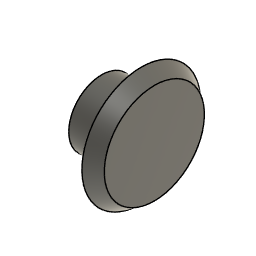
Four-Cylinder Engine_ (Autodesk Fusion 360 archive; units mm, degrees)
design "Rivet"
Autodesk Fusion 360 part; units mm, degrees
sketch "Sketch1" plane through (0, 0, 0) normal (0, 1, 0) x (1, 0, 0)
  line L0 (0, 0) -> (101.6, 0)
  line L1 (101.6, 0) -> (101.6, -96.5147)
  line L2 (101.6, -96.5147) -> (76.2, -114.3)
  line L3 (76.2, -114.3) -> (76.2, -63.5)
  line L4 (76.2, -63.5) -> (0, -63.5)
  line L5 (0, -63.5) -> (0, 0)
  dimension "d1" = 101.6
  dimension "d2" = 76.2
  dimension "d3" = 55
  dimension "d4" = 127
  dimension "d5" = 228.6
  constraint coincident L0.start L5.end
  constraint horizontal L0
  constraint perpendicular L0 L3
  constraint perpendicular L3 L4
  constraint vertical L1
  constraint vertical L5
  measures "d1" distance of L0.start L0.end
  measures "d2" distance of L3.end L4.end
  measures "d3" angle of L2 L3
revolve "Revolve1" add sketch "Sketch1" angle 360 about axis through (0, 0, 0) along (1, 0, 0)

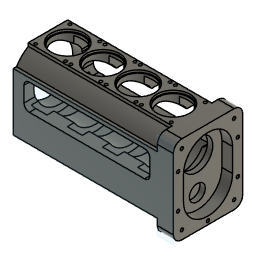
design "Engine Block"
Autodesk Fusion 360 part; units mm, degrees
sketch "Sketch1" plane through (0, 0, 0) normal (1, 0, 0) x (0, 1, 0)
  line L0 (-825.5, 1041.4) -> (825.5, 1041.4)
  line L1 (825.5, 1041.4) -> (825.5, -1041.4)
  line L2 (825.5, -1041.4) -> (-825.5, -1041.4)
  line L3 (-825.5, -1041.4) -> (-825.5, 1041.4)
  line L4 (-825.5, 1041.4) -> (825.5, -1041.4) construction
  line L5 (825.5, 1041.4) -> (-825.5, -1041.4) construction
  dimension "d1" = 1651
  dimension "d2" = 2082.8
  constraint horizontal L0
  constraint perpendicular L0 L1
  constraint parallel L0 L2
  constraint parallel L1 L3
  constraint coincident L4 origin
  constraint coincident L5 origin
  measures "d1" distance of L0.start L0.end
  measures "d2" distance of L0.end L1.end
extrude "Extrude1" add sketch "Sketch1" along normal mid plane 3810
sketch "Sketch2" plane through (1905, 0, 0) normal (1, 0, 0) x (0, 1, 0)
  line L0 (-825.5, -1041.4) -> (825.5, -1041.4)
  line L1 (825.5, -1041.4) -> (825.5, 1041.4)
  line L2 (825.5, 1041.4) -> (-825.5, 1041.4)
  line L3 (-825.5, 1041.4) -> (-825.5, -1041.4)
  circle A0 centre (0, 279.4) radius 368.3
  dimension "d5" = 736.6
  dimension "d6" = 279.4
  constraint vertical origin A0.centre
  measures "d5" diameter of A0
  measures "d6" distance of origin A0.centre
extrude "Extrude2" cut sketch "Sketch2" against normal through all contours A0
sketch "Sketch3" plane through (1905, 0, 0) normal (1, 0, 0) x (0, 1, 0)
  circle A0 centre (0, 279.4) radius 368.3
  line L0 (-825.5, -1041.4) -> (825.5, -1041.4)
  line L1 (825.5, -1041.4) -> (825.5, 1041.4)
  line L2 (825.5, 1041.4) -> (-825.5, 1041.4)
  line L3 (-825.5, 1041.4) -> (-825.5, -1041.4)
  line L4 (-584.2, 279.4) -> (-584.2, -279.4)
  arc A1 (-584.2, -279.4) -> (584.2, -279.4) centre (0, -279.4) ccw
  line L5 (584.2, -279.4) -> (584.2, 279.4)
  arc A2 (584.2, 279.4) -> (-584.2, 279.4) centre (0, 279.4) ccw
  line L6 (0, 279.4) -> (0, -279.4) construction
  dimension "d8" = 584.2
  dimension "d9" = 558.8
  constraint tangent L4 A1
  constraint tangent A1 L5
  constraint parallel L4 L5
  constraint tangent L5 A2
  constraint tangent L4 A2
  constraint vertical L6
  constraint coincident A0.centre A2.centre
  measures "d8" radius of A2
  measures "d9" distance of A0.centre A1.centre
extrude "Extrude3" cut sketch "Sketch3" against normal blind 254 contours L4 A1 L5 A2
sketch "Sketch4" plane through (-1905, 0, 0) normal (-1, 0, 0) x (0, -1, 0)
  circle A0 centre (0, 279.4) radius 368.3
  line L0 (-825.5, -1041.4) -> (825.5, -1041.4)
  line L1 (825.5, -1041.4) -> (825.5, 1041.4)
  line L2 (825.5, 1041.4) -> (-825.5, 1041.4)
  line L3 (-825.5, 1041.4) -> (-825.5, -1041.4)
  circle A1 centre (0, 279.4) radius 590.55
  dimension "d12" = 1181.1
  constraint concentric A0 A1
  measures "d12" diameter of A1
extrude "Extrude4" cut sketch "Sketch4" against normal blind 3429 contours A1
sketch "Sketch5" plane through (-1905, 0, 0) normal (-1, 0, 0) x (0, -1, 0)
  circle A0 centre (0, 279.4) radius 590.55
  line L0 (-825.5, -1041.4) -> (825.5, -1041.4)
  line L1 (825.5, -1041.4) -> (825.5, 1041.4)
  line L2 (825.5, 1041.4) -> (-825.5, 1041.4)
  line L3 (-825.5, 1041.4) -> (-825.5, -1041.4)
  line L4 (-419.1, -1041.4) -> (-749.3, -685.8)
  line L5 (-749.3, -685.8) -> (-825.5, -685.8)
  line L6 (-825.5, 685.8) -> (-749.3, 685.8)
  line L7 (-469.9, 965.2) -> (-469.9, 1041.4)
  line L8 (0, 0) -> (0, 1263.6507) construction
  arc A1 (-469.9, 965.2) -> (-749.3, 685.8) centre (-15.1369, 231.0369) ccw
  line L9 (825.5, 685.8) -> (749.3, 685.8)
  arc A2 (749.3, 685.8) -> (469.9, 965.2) centre (15.1369, 231.0369) ccw
  line L10 (469.9, 965.2) -> (469.9, 1041.4)
  line L11 (749.3, -685.8) -> (825.5, -685.8)
  line L12 (419.1, -1041.4) -> (749.3, -685.8)
  dimension "d15" = 76.2
  dimension "d16" = 76.2
  dimension "d17" = 355.6
  dimension "d18" = 355.6
  dimension "d20" = 863.6
  dimension "d21" = 76.2
  dimension "d22" = 355.6
  dimension "d23" = 406.4
  constraint coincident L0 L4.start
  constraint coincident L3 L5.end
  constraint perpendicular L3 L5
  constraint coincident L3 L6.start
  constraint perpendicular L3 L6
  constraint coincident L2 L7.end
  constraint perpendicular L2 L7
  constraint coincident L8.start origin
  constraint perpendicular L2 L8
  constraint symmetric L4.start L8 L12.start
  constraint symmetric L4.end L8 L11.start
  constraint symmetric L5.end L8 L11.end
  constraint symmetric L6.start L8 L9.start
  constraint symmetric L6.end L8 L9.end
  constraint symmetric L7.start L8 A2.end
  constraint symmetric L7.end L8 L10.end
  constraint symmetric L8 A1 A2
  measures "d15" distance of L7.start L7.end
  measures "d16" distance of L6.start L6.end
  measures "d17" distance of L2.end L7.end
  measures "d18" distance of L2.end L6.start
  measures "d20" radius of A1
  measures "d21" distance of L4.end L5.end
  measures "d22" distance of L0.start L5.end
  measures "d23" distance of L0.start L4.start
extrude "Extrude5" cut sketch "Sketch5" against normal blind 3429 contours L0 L3 L4 L5 | L0 L1 L11 L12 | L2 L3 L6 L7 A1 | L1 L2 L9 A2 L10
sketch "Sketch6" plane through (0, 0, 1041.4) normal (0, 0, 1) x (-1, 0, 0)
  line L0 (-1524, 469.9) -> (-1524, 825.5)
  line L1 (-1524, 825.5) -> (-1905, 825.5)
  line L2 (-1905, 825.5) -> (-1905, -825.5)
  line L3 (-1905, -825.5) -> (-1524, -825.5)
  line L4 (-1524, -825.5) -> (-1524, -469.9)
  line L5 (-1524, -469.9) -> (1905, -469.9)
  line L6 (1905, -469.9) -> (1905, 469.9)
  line L7 (1905, 469.9) -> (-1524, 469.9)
  circle A0 centre (-1079.5, 0) radius 368.3
  circle A1 centre (-241.3, 0) radius 368.3
  circle A2 centre (596.9, 0) radius 368.3
  circle A3 centre (1435.1, 0) radius 368.3
  dimension "d26" = 736.6
  dimension "d27" = 825.5
  dimension "d30" = 2514.6
  dimension "d31" = 0
  constraint horizontal origin A0.centre
  measures "d26" diameter of A0
  measures "d27" distance of L2 A0.centre
extrude "Extrude6" cut sketch "Sketch6" against normal blind 762 contours A0 | A1 | A2 | A3
sketch "Sketch7" plane through (0, 0, 1041.4) normal (0, 0, 1) x (-1, 0, 0)
  circle A0 centre (596.9, 0) radius 368.3
  circle A1 centre (-241.3, 0) radius 368.3
  circle A2 centre (1435.1, 0) radius 368.3
  circle A3 centre (-1079.5, 0) radius 368.3
  line L0 (-1524, 469.9) -> (-1524, 825.5)
  line L1 (-1524, 825.5) -> (-1905, 825.5)
  line L2 (-1905, 825.5) -> (-1905, -825.5)
  line L3 (-1905, -825.5) -> (-1524, -825.5)
  line L4 (-1524, -825.5) -> (-1524, -469.9)
  line L5 (-1524, -469.9) -> (1905, -469.9)
  line L6 (1905, -469.9) -> (1905, 469.9)
  line L7 (1905, 469.9) -> (-1524, 469.9)
  circle A4 centre (-1079.5, 0) radius 393.7
  circle A5 centre (-241.3, 0) radius 393.7
  circle A6 centre (596.9, 0) radius 393.7
  circle A7 centre (1435.1, 0) radius 393.7
  dimension "d34" = 787.4
  dimension "d37" = 2514.6
  dimension "d38" = 0
  constraint concentric A3 A4
  measures "d34" diameter of A4
extrude "Extrude7" cut sketch "Sketch7" against normal blind 50.8 contours A4 | A5 | A6 | A7
sketch "Sketch8" plane through (0, -825.5, 0) normal (0, -1, 0) x (1, 0, 0)
  line L0 (1524, 1041.4) -> (1524, 685.8)
  line L1 (1524, 685.8) -> (-1905, 685.8)
  line L2 (-1905, 685.8) -> (-1905, -685.8)
  line L3 (-1905, -685.8) -> (1524, -685.8)
  line L4 (1524, -685.8) -> (1524, -1041.4)
  line L5 (1524, -1041.4) -> (1905, -1041.4)
  line L6 (1905, -1041.4) -> (1905, 1041.4)
  line L7 (1905, 1041.4) -> (1524, 1041.4)
sketch "Sketch9" plane through (0, 0, 0) normal (0, 1, 0) x (1, 0, 0)
  line L0 (-2322.3907, -279.4) -> (2570.9498, -279.4) construction
  line L1 (901.7, -1016) -> (1257.3, -1016)
  line L2 (1257.3, -1016) -> (1257.3, -279.4)
  line L3 (1257.3, -279.4) -> (901.7, -279.4)
  line L4 (901.7, -279.4) -> (901.7, -1016)
  point P0 (1905, -1041.4)
  dimension "d41" = 355.6
  dimension "d42" = 647.7
  dimension "d43" = 1473.2
  dimension "d44" = 279.4
  constraint horizontal L0
  constraint horizontal L1
  constraint vertical L2
  constraint horizontal L3
  constraint vertical L4
  constraint coincident L0 L2.end
  measures "d41" distance of L1.start L1.end
  measures "d42" horizontal distance of L1.end P0
  measures "d44" distance of L0 origin
revolve "Revolve1" cut sketch "Sketch9" angle 360 about axis through (-2322.3907, 0, 279.4) along (1, 0, 0)
pattern_linear "R-Pattern1" count 4 spacing 838.2 along (-1, 0, 0) of "Revolve1"
sketch "Sketch10" plane through (0, -825.5, 0) normal (0, -1, 0) x (1, 0, 0)
  line L0 (-1524, 596.9) -> (1219.2, 596.9)
  line L1 (1346.2, 469.9) -> (1346.2, 101.6)
  line L2 (1219.2, -25.4) -> (-1524, -25.4)
  line L3 (-1651, 101.6) -> (-1651, 469.9)
  arc A0 (1346.2, 469.9) -> (1219.2, 596.9) centre (1219.2, 469.9) ccw
  arc A1 (1219.2, -25.4) -> (1346.2, 101.6) centre (1219.2, 101.6) ccw
  arc A2 (-1651, 101.6) -> (-1524, -25.4) centre (-1524, 101.6) ccw
  arc A3 (-1524, 596.9) -> (-1651, 469.9) centre (-1524, 469.9) ccw
  point P0 (-1651, 596.9)
  point P1 (1346.2, 596.9)
  point P2 (1346.2, -25.4)
  point P3 (1905, 1041.4)
  point P4 (-1905, 1041.4)
  point P5 (1905, -1041.4)
  dimension "d50" = 558.8
  dimension "d51" = 444.5
  dimension "d52" = 254
  dimension "d53" = 1016
  dimension "d54" = 127
  constraint horizontal L0
  constraint vertical L1
  constraint horizontal L2
  constraint vertical L3
  constraint coincident P1 L0
  constraint coincident P1 L1
  constraint tangent L0 A0
  constraint tangent L1 A0
  constraint coincident P2 L1
  constraint coincident P2 L2
  constraint tangent L1 A1
  constraint tangent L2 A1
  constraint equal A0 A1
  constraint tangent L2 A2
  constraint tangent L3 A2
  constraint equal A0 A2
  constraint coincident P0 L0
  constraint coincident P0 L3
  constraint tangent L0 A3
  constraint tangent L3 A3
  constraint equal A0 A3
  measures "d50" horizontal distance of P1 P3
  measures "d51" vertical distance of P1 P3
  measures "d52" horizontal distance of P0 P4
  measures "d53" vertical distance of P2 P5
  measures "d54" radius of A0
extrude "Extrude8" cut sketch "Sketch10" against normal blind 2540
sketch "Sketch11" plane through (0, 0, 1041.4) normal (0, 0, 1) x (-1, 0, 0)
  circle A0 centre (-241.3, 0) radius 393.7
  circle A1 centre (596.9, 0) radius 393.7
  circle A2 centre (-1079.5, 0) radius 393.7
  circle A3 centre (1435.1, 0) radius 393.7
  line L0 (-1524, 469.9) -> (-1524, 825.5)
  line L1 (-1524, 825.5) -> (-1905, 825.5)
  line L2 (-1905, 825.5) -> (-1905, -825.5)
  line L3 (-1905, -825.5) -> (-1524, -825.5)
  line L4 (-1524, -825.5) -> (-1524, -469.9)
  line L5 (-1524, -469.9) -> (1905, -469.9)
  line L6 (1905, -469.9) -> (1905, 469.9)
  line L7 (1905, 469.9) -> (-1524, 469.9)
  line L8 (-1435.1, 406.4) -> (-723.9, 406.4) construction
  line L9 (-723.9, 406.4) -> (-723.9, -406.4) construction
  line L10 (-723.9, -406.4) -> (-1435.1, -406.4) construction
  line L11 (-1435.1, -406.4) -> (-1435.1, 406.4) construction
  line L12 (-1435.1, 406.4) -> (-723.9, -406.4) construction
  line L13 (-723.9, 406.4) -> (-1435.1, -406.4) construction
  point P0 (-1079.5, 0)
  dimension "d57" = 711.2
  dimension "d58" = 812.8
  constraint horizontal L8
  constraint perpendicular L8 L9
  constraint parallel L8 L10
  constraint parallel L9 L11
  constraint coincident L12 P0
  constraint coincident L13 P0
  constraint coincident P0 A2.centre
  measures "d57" distance of L9.end L10.end
  measures "d58" distance of L8.start L10.end
hole "Hole1" at (723.9, 406.4, 1041.4) at (1435.1, 406.4, 1041.4) at (1435.1, -406.4, 1041.4) at (723.9, -406.4, 1041.4) direction (0, 0, -1) diameter 69.85 depth 127 tip angle 118
pattern_linear "R-Pattern2" count 4 spacing 838.2 along (-1, 0, 0) of "Hole1"
sketch "Sketch12" plane through (1651, 0, 0) normal (1, 0, 0) x (0, 1, 0)
  circle A0 centre (0, 279.4) radius 368.3
  arc A1 (584.2, 279.4) -> (-584.2, 279.4) centre (0, 279.4) ccw
  line L0 (-584.2, 279.4) -> (-584.2, -279.4)
  arc A2 (-584.2, -279.4) -> (584.2, -279.4) centre (0, -279.4) ccw
  line L1 (584.2, -279.4) -> (584.2, 279.4)
  circle A3 centre (0, -508) radius 190.5
  dimension "d66" = 381
  dimension "d67" = 508
  constraint vertical origin A3.centre
  measures "d66" diameter of A3
  measures "d67" distance of origin A3.centre
extrude "Extrude9" cut sketch "Sketch12" against normal blind 127 contours A3
sketch "Sketch13" plane through (1905, 0, 0) normal (1, 0, 0) x (0, 1, 0)
  line L0 (-584.2, -279.4) -> (-584.2, 279.4)
  arc A0 (584.2, 279.4) -> (-584.2, 279.4) centre (0, 279.4) ccw
  line L1 (584.2, 279.4) -> (584.2, -279.4)
  arc A1 (-584.2, -279.4) -> (584.2, -279.4) centre (0, -279.4) ccw
  line L2 (-825.5, -1041.4) -> (825.5, -1041.4)
  line L3 (825.5, -1041.4) -> (825.5, 1041.4)
  line L4 (825.5, 1041.4) -> (-825.5, 1041.4)
  line L5 (-825.5, 1041.4) -> (-825.5, -1041.4)
  line L6 (0, 0) -> (0, 1187.2855) construction
  line L7 (-825.5, -1041.4) -> (-825.5, 1041.4)
  point P0 (-622.3, 838.2)
  point P1 (-711.2, 406.4)
  point P2 (-711.2, -406.4)
  point P3 (-622.3, -838.2)
  point P4 (0, -960.12)
  point P5 (622.3, 838.2)
  point P6 (711.2, 406.4)
  point P7 (711.2, -406.4)
  point P8 (622.3, -838.2)
  point P9 (0, -960.12)
  dimension "d70" = 203.2
  dimension "d71" = 711.2
  dimension "d72" = 431.8
  dimension "d73" = 406.4
  dimension "d74" = 812.8
  dimension "d75" = 431.8
  dimension "d76" = 960.12
  dimension "d77" = 203.2
  constraint coincident L6.start origin
  constraint perpendicular L4 L6
  constraint vertical P1 P2
  constraint vertical L6.start P9
  constraint symmetric L6 P0 P5
  constraint symmetric L6 P1 P6
  constraint symmetric L6 P2 P7
  constraint symmetric L6 P3 P8
  constraint symmetric L6 P9 P4
  measures "d70" distance of P0 L7
  measures "d71" distance of L6 P1
  measures "d72" vertical distance of P0 P1
  measures "d73" vertical distance of L6.start P1
  measures "d74" vertical distance of P1 P2
  measures "d75" vertical distance of P2 P3
  measures "d76" distance of L6.start P9
  measures "d77" horizontal distance of P3 L2.start
hole "Hole2" at (1905, -622.3, 838.2) at (1905, -711.2, 406.4) at (1905, -711.2, -406.4) at (1905, -622.3, -838.2) at (1905, 0, -960.12) at (1905, 622.3, -838.2) at (1905, 711.2, -406.4) at (1905, 711.2, 406.4) at (1905, 622.3, 838.2) direction (-1, 0, 0) diameter 68.58 depth 127 tip angle 118 countersink diameter 76.2 countersink angle 82
fillet "Fillet1" radius 203.2 4 edges at (1714.5, -825.5, 1041.4) (1714.5, 825.5, 1041.4) (1714.5, 825.5, -1041.4) (1714.5, -825.5, -1041.4)

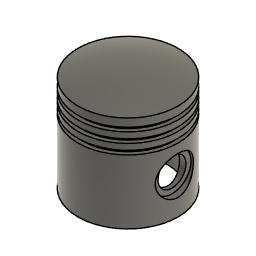
design "Piston"
Autodesk Fusion 360 part; units mm, degrees
sketch "Sketch1" plane through (0, 0, 0) normal (0, 1, 0) x (1, 0, 0)
  line L0 (0, 0) -> (0, -408.4277) construction
  line L1 (0, -660.4) -> (0, -355.6)
  line L2 (0, -355.6) -> (254, -355.6)
  line L3 (254, -355.6) -> (254, 0)
  line L4 (254, 0) -> (317.5, 0)
  line L5 (317.5, 0) -> (317.5, -406.4)
  line L6 (317.5, -406.4) -> (292.1, -406.4)
  line L7 (292.1, -406.4) -> (292.1, -431.8)
  line L8 (292.1, -431.8) -> (317.5, -431.8)
  line L9 (317.5, -431.8) -> (317.5, -469.9)
  line L10 (317.5, -469.9) -> (292.1, -469.9)
  line L11 (292.1, -469.9) -> (292.1, -495.3)
  line L12 (292.1, -495.3) -> (317.5, -495.3)
  line L13 (317.5, -495.3) -> (317.5, -533.4)
  line L14 (317.5, -533.4) -> (292.1, -533.4)
  line L15 (292.1, -533.4) -> (292.1, -558.8)
  line L16 (292.1, -558.8) -> (317.5, -558.8)
  line L17 (317.5, -558.8) -> (317.5, -609.6)
  arc A0 (0, -660.4) -> (317.5, -609.6) centre (0, 357.1875) ccw
  line L18 (0, -660.4) -> (-298.2009, -660.4) construction
  dimension "d1" = 508
  dimension "d2" = 635
  dimension "d3" = 355.6
  dimension "d4" = 406.4
  dimension "d5" = 25.4
  dimension "d6" = 25.4
  dimension "d7" = 38.1
  dimension "d8" = 50.8
  dimension "d9" = 660.4
  constraint coincident L0.start origin
  constraint vertical L0
  constraint coincident L0 L1.start
  constraint coincident L0 L1.end
  constraint perpendicular L1 L2
  constraint perpendicular L2 L3
  constraint perpendicular L0 L4
  constraint perpendicular L4 L5
  constraint perpendicular L5 L6
  constraint perpendicular L6 L7
  constraint perpendicular L7 L8
  constraint perpendicular L8 L9
  constraint perpendicular L9 L10
  constraint perpendicular L10 L11
  constraint perpendicular L11 L12
  constraint perpendicular L12 L13
  constraint perpendicular L13 L14
  constraint perpendicular L14 L15
  constraint perpendicular L15 L16
  constraint perpendicular L16 L17
  constraint horizontal L0.start L3.end
  constraint vertical L5.end L8.end
  constraint vertical L9.end L12.end
  constraint vertical L13.end L17.end
  constraint equal L7 L11
  constraint equal L11 L15
  constraint equal L9 L13
  constraint vertical L7.end L10.end
  constraint vertical L11.end L14.end
  constraint perpendicular L1 L18
  constraint tangent A0 L18
  measures "d3" distance of L2.end L3.end
  measures "d4" distance of L4.end L5.end
  measures "d5" distance of L5.end L6.end
  measures "d6" distance of L6.end L7.end
  measures "d7" distance of L8.end L9.end
  measures "d8" distance of L16.end L17.end
  measures "d9" distance of L0.start L1.start
revolve "Revolve1" add sketch "Sketch1" angle 360 about axis through (0, 0, 0) along (0, 0, 1)
ref_plane "WorkPlane1" through (317.5, 0, 0) normal (1, 0, 0) x (0, 1, 0)
sketch "Sketch2" plane through (317.5, 0, 0) normal (1, 0, 0) x (0, 1, 0)
  circle A0 centre (0, 228.6) radius 120.65
  dimension "d12" = 241.3
  dimension "d13" = 228.6
  constraint vertical origin A0.centre
  measures "d12" diameter of A0
  measures "d13" distance of origin A0.centre
extrude "Extrude1" cut sketch "Sketch2" against normal blind 38.1
sketch "Sketch3" plane through (279.4, 0, 0) normal (1, 0, 0) x (0, 1, 0)
  circle A0 centre (0, 228.6) radius 120.65
  circle A1 centre (0, 228.6) radius 88.9
  dimension "d16" = 177.8
  constraint concentric A0 A1
  measures "d16" diameter of A1
extrude "Extrude2" cut sketch "Sketch3" against normal blind 127 contours A1
mirror "Mirror1" about plane through (0, 0, 0) normal (1, 0, 0) of "Extrude1", "Extrude2"

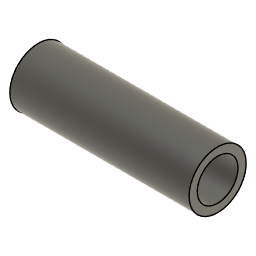
design "Piston Pin"
Autodesk Fusion 360 part; units mm, degrees
sketch "Sketch1" plane through (0, 0, 0) normal (1, 0, 0) x (0, 1, 0)
  circle A0 centre (0, 0) radius 63.5
  circle A1 centre (0, 0) radius 88.9
  dimension "d1" = 127
  dimension "d2" = 177.8
  constraint coincident A0.centre A1.centre
  constraint concentric A0 A1
  measures "d1" diameter of A0
  measures "d2" diameter of A1
extrude "Extrude1" add sketch "Sketch1" along normal blind 558.8

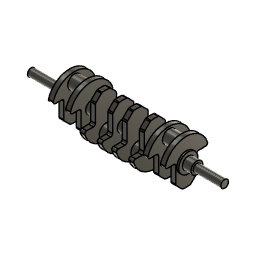
design "Crankshaft"
Autodesk Fusion 360 part; units mm, degrees
sketch "Sketch1" plane through (0, 0, 0) normal (0, 1, 0) x (1, 0, 0)
  line L0 (0, 0) -> (1016, 0)
  line L1 (1016, 0) -> (1016, -254)
  line L2 (1016, -254) -> (965.2, -254)
  line L3 (965.2, -254) -> (965.2, -158.75)
  line L4 (965.2, -158.75) -> (736.6, -158.75)
  line L5 (736.6, -158.75) -> (736.6, -101.6)
  line L6 (736.6, -101.6) -> (0, -101.6)
  line L7 (0, -101.6) -> (0, 0)
  dimension "d1" = 1016
  dimension "d2" = 203.2
  dimension "d3" = 317.5
  dimension "d4" = 508
  dimension "d5" = 50.8
  dimension "d6" = 228.6
  constraint coincident L0.start L7.end
  constraint horizontal L0
  constraint perpendicular L0 L1
  constraint perpendicular L1 L2
  constraint perpendicular L2 L3
  constraint perpendicular L3 L4
  constraint perpendicular L4 L5
  constraint perpendicular L5 L6
  constraint perpendicular L0 L7
  measures "d1" distance of L0.start L0.end
  measures "d5" distance of L1.end L2.end
  measures "d6" distance of L3.end L4.end
revolve "Revolve1" add sketch "Sketch1" angle 360 about axis through (0, 0, 0) along (1, 0, 0)
sketch "Sketch2" plane through (1016, 0, 0) normal (1, 0, 0) x (0, 1, 0)
  circle A0 centre (0, 0) radius 254
  line L0 (-575.2974, 101.6) -> (-279.4, 101.6)
  line L1 (-279.4, 101.6) -> (-279.4, -406.4)
  line L2 (-279.4, -406.4) -> (-112.5429, -573.2571)
  line L3 (0, 0) -> (0, -701.9351) construction
  line L4 (279.4, -406.4) -> (112.5429, -573.2571)
  line L5 (279.4, 101.6) -> (279.4, -406.4)
  line L6 (575.2974, 101.6) -> (279.4, 101.6)
  arc A1 (575.2974, 101.6) -> (-575.2974, 101.6) centre (0, 0) ccw
  arc A2 (-112.5429, -573.2571) -> (112.5429, -573.2571) centre (0, 0) ccw
  dimension "d8" = 1168.4
  dimension "d9" = 101.6
  dimension "d10" = 135
  dimension "d11" = 508
  dimension "d12" = 558.8
  constraint concentric A0 A1
  constraint horizontal L0
  constraint perpendicular L0 L1
  constraint coincident L2.end A1
  constraint coincident A0.centre L3.start
  constraint vertical L3
  constraint symmetric L0.start L3 L6.start
  constraint symmetric L0.end L3 L5.start
  constraint symmetric L1.end L3 L4.start
  constraint symmetric L2.end L3 L4.end
  constraint concentric A1 A2
  measures "d8" diameter of A1
  measures "d9" distance of A0.centre L0
  measures "d10" angle of L1 L2
  measures "d11" distance of L0.end L1.end
  measures "d12" distance of L1 L5
extrude "Extrude1" add sketch "Sketch2" along normal blind 127 contours A0 | L0 L1 L2 L4 L5 L6 A1 A2
fillet "Fillet1" radius 50.8 8 edges at (1079.5, 575.2974, 101.6) (1079.5, 279.4, 101.6) (1079.5, 279.4, -406.4) (1079.5, 112.5429, -573.2571) (1079.5, -112.5429, -573.2571) (1079.5, -279.4, -406.4) (1079.5, -279.4, 101.6) (1079.5, -575.2974, 101.6)
sketch "Sketch3" plane through (1143, 0, 0) normal (1, 0, 0) x (0, 1, 0)
  arc A0 (-559.8475, 166.9143) -> (-511.1651, 101.6) centre (-511.1651, 152.4) ccw
  line L0 (-511.1651, 101.6) -> (-330.2, 101.6)
  arc A1 (-279.4, 50.8) -> (-330.2, 101.6) centre (-330.2, 50.8) ccw
  line L1 (-279.4, 50.8) -> (-279.4, -385.358)
  arc A2 (-279.4, -385.358) -> (-264.521, -421.279) centre (-228.6, -385.358) ccw
  line L2 (-264.521, -421.279) -> (-123.7615, -562.0385)
  arc A3 (-123.7615, -562.0385) -> (-96.2062, -576.2239) centre (-87.8405, -526.1175) ccw
  arc A4 (-96.2062, -576.2239) -> (96.2062, -576.2239) centre (0, 0) ccw
  arc A5 (96.2062, -576.2239) -> (123.7615, -562.0385) centre (87.8405, -526.1175) ccw
  line L3 (123.7615, -562.0385) -> (264.521, -421.279)
  arc A6 (264.521, -421.279) -> (279.4, -385.358) centre (228.6, -385.358) ccw
  line L4 (279.4, -385.358) -> (279.4, 50.8)
  arc A7 (330.2, 101.6) -> (279.4, 50.8) centre (330.2, 50.8) ccw
  line L5 (330.2, 101.6) -> (511.1651, 101.6)
  arc A8 (511.1651, 101.6) -> (559.8475, 166.9143) centre (511.1651, 152.4) ccw
  arc A9 (559.8475, 166.9143) -> (-559.8475, 166.9143) centre (0, 0) ccw
  circle A10 centre (0, 355.6) radius 177.8
  dimension "d17" = 355.6
  dimension "d18" = 355.6
  constraint vertical A4.centre A10.centre
  measures "d17" diameter of A10
  measures "d18" distance of A4.centre A10.centre
extrude "Extrude2" add sketch "Sketch3" along normal blind 330.2 contours A10
pattern_linear "R-Pattern1" count 2 spacing 457.2 along (1, 0, 0) of "Extrude1", "Fillet1"
sketch "Sketch4" plane through (1600.2, 0, 0) normal (1, 0, 0) x (0, 1, 0)
  arc A0 (-559.8475, 166.9143) -> (-511.1651, 101.6) centre (-511.1651, 152.4) ccw
  line L0 (-511.1651, 101.6) -> (-330.2, 101.6)
  arc A1 (-279.4, 50.8) -> (-330.2, 101.6) centre (-330.2, 50.8) ccw
  line L1 (-279.4, 50.8) -> (-279.4, -385.358)
  arc A2 (-279.4, -385.358) -> (-264.521, -421.279) centre (-228.6, -385.358) ccw
  line L2 (-264.521, -421.279) -> (-123.7615, -562.0385)
  arc A3 (-123.7615, -562.0385) -> (-96.2062, -576.2239) centre (-87.8405, -526.1175) ccw
  arc A4 (-96.2062, -576.2239) -> (96.2062, -576.2239) centre (0, 0) ccw
  arc A5 (96.2062, -576.2239) -> (123.7615, -562.0385) centre (87.8405, -526.1175) ccw
  line L3 (123.7615, -562.0385) -> (264.521, -421.279)
  arc A6 (264.521, -421.279) -> (279.4, -385.358) centre (228.6, -385.358) ccw
  line L4 (279.4, -385.358) -> (279.4, 50.8)
  arc A7 (330.2, 101.6) -> (279.4, 50.8) centre (330.2, 50.8) ccw
  line L5 (330.2, 101.6) -> (511.1651, 101.6)
  arc A8 (511.1651, 101.6) -> (559.8475, 166.9143) centre (511.1651, 152.4) ccw
  arc A9 (559.8475, 166.9143) -> (-559.8475, 166.9143) centre (0, 0) ccw
  circle A10 centre (0, 0) radius 158.75
  dimension "d25" = 317.5
  constraint coincident A4.centre A9.centre
  measures "d25" diameter of A10
extrude "Extrude3" add sketch "Sketch4" along normal blind 254 contours A10
sketch "Sketch5" plane through (1854.2, 0, 0) normal (1, 0, 0) x (0, 1, 0)
  circle A0 centre (0, 0) radius 158.75
  line L0 (-575.2974, -101.6) -> (-279.4, -101.6)
  line L1 (-279.4, -101.6) -> (-279.4, 406.4)
  line L2 (-279.4, 406.4) -> (-112.5429, 573.2571)
  line L3 (0, 0) -> (0, 823.9979) construction
  line L4 (575.2974, -101.6) -> (279.4, -101.6)
  line L5 (279.4, -101.6) -> (279.4, 406.4)
  line L6 (279.4, 406.4) -> (112.5429, 573.2571)
  arc A1 (-575.2974, -101.6) -> (575.2974, -101.6) centre (0, 0) ccw
  arc A2 (112.5429, 573.2571) -> (-112.5429, 573.2571) centre (0, 0) ccw
  dimension "d28" = 1168.4
  dimension "d29" = 135
  dimension "d30" = 508
  dimension "d31" = 279.4
  dimension "d32" = 101.6
  dimension "d33" = 584.2
  constraint concentric A0 A1
  constraint horizontal L0
  constraint perpendicular L0 L1
  constraint coincident A0.centre L3.start
  constraint parallel L1 L3
  constraint symmetric L0.start L3 L4.start
  constraint symmetric L0.end L3 L4.end
  constraint symmetric L1.end L3 L5.end
  constraint symmetric L2.end L3 L6.end
  constraint concentric A1 A2
  measures "d28" diameter of A1
  measures "d29" angle of L1 L2
  measures "d30" distance of L0.end L1.end
  measures "d31" distance of L1 L3
  measures "d32" distance of A0.centre L0
  measures "d33" radius of A2
extrude "Extrude4" add sketch "Sketch5" along normal blind 127 contours A0 | L0 L1 L2 L4 L5 L6 A1 A2
fillet "Fillet2" radius 50.8 8 edges at (1917.7, -279.4, -101.6) (1917.7, -575.2974, -101.6) (1917.7, -279.4, 406.4) (1917.7, -112.5429, 573.2571) (1917.7, 112.5429, 573.2571) (1917.7, 279.4, 406.4) (1917.7, 279.4, -101.6) (1917.7, 575.2974, -101.6)
sketch "Sketch6" plane through (1981.2, 0, 0) normal (1, 0, 0) x (0, 1, 0)
  arc A0 (559.8475, -166.9143) -> (511.1651, -101.6) centre (511.1651, -152.4) ccw
  line L0 (511.1651, -101.6) -> (330.2, -101.6)
  arc A1 (279.4, -50.8) -> (330.2, -101.6) centre (330.2, -50.8) ccw
  line L1 (279.4, -50.8) -> (279.4, 385.358)
  arc A2 (279.4, 385.358) -> (264.521, 421.279) centre (228.6, 385.358) ccw
  line L2 (264.521, 421.279) -> (123.7615, 562.0385)
  arc A3 (123.7615, 562.0385) -> (96.2062, 576.2239) centre (87.8405, 526.1175) ccw
  arc A4 (96.2062, 576.2239) -> (-96.2062, 576.2239) centre (0, 0) ccw
  arc A5 (-96.2062, 576.2239) -> (-123.7615, 562.0385) centre (-87.8405, 526.1175) ccw
  line L3 (-123.7615, 562.0385) -> (-264.521, 421.279)
  arc A6 (-264.521, 421.279) -> (-279.4, 385.358) centre (-228.6, 385.358) ccw
  line L4 (-279.4, 385.358) -> (-279.4, -50.8)
  arc A7 (-330.2, -101.6) -> (-279.4, -50.8) centre (-330.2, -50.8) ccw
  line L5 (-330.2, -101.6) -> (-511.1651, -101.6)
  arc A8 (-511.1651, -101.6) -> (-559.8475, -166.9143) centre (-511.1651, -152.4) ccw
  arc A9 (-559.8475, -166.9143) -> (559.8475, -166.9143) centre (0, 0) ccw
  circle A10 centre (0, -355.6) radius 177.8
  dimension "d38" = 355.6
  dimension "d39" = 355.6
  constraint vertical A4.centre A10.centre
  measures "d38" diameter of A10
  measures "d39" distance of A4.centre A10.centre
extrude "Extrude5" add sketch "Sketch6" along normal blind 330.2 contours A10
pattern_linear "R-Pattern2" count 2 spacing 457.2 along (1, 0, 0) of "Extrude4", "Fillet2"
sketch "Sketch7" plane through (2438.4, 0, 0) normal (1, 0, 0) x (0, 1, 0)
  arc A0 (559.8475, -166.9143) -> (511.1651, -101.6) centre (511.1651, -152.4) ccw
  line L0 (511.1651, -101.6) -> (330.2, -101.6)
  arc A1 (279.4, -50.8) -> (330.2, -101.6) centre (330.2, -50.8) ccw
  line L1 (279.4, -50.8) -> (279.4, 385.358)
  arc A2 (279.4, 385.358) -> (264.521, 421.279) centre (228.6, 385.358) ccw
  line L2 (264.521, 421.279) -> (123.7615, 562.0385)
  arc A3 (123.7615, 562.0385) -> (96.2062, 576.2239) centre (87.8405, 526.1175) ccw
  arc A4 (96.2062, 576.2239) -> (-96.2062, 576.2239) centre (0, 0) ccw
  arc A5 (-96.2062, 576.2239) -> (-123.7615, 562.0385) centre (-87.8405, 526.1175) ccw
  line L3 (-123.7615, 562.0385) -> (-264.521, 421.279)
  arc A6 (-264.521, 421.279) -> (-279.4, 385.358) centre (-228.6, 385.358) ccw
  line L4 (-279.4, 385.358) -> (-279.4, -50.8)
  arc A7 (-330.2, -101.6) -> (-279.4, -50.8) centre (-330.2, -50.8) ccw
  line L5 (-330.2, -101.6) -> (-511.1651, -101.6)
  arc A8 (-511.1651, -101.6) -> (-559.8475, -166.9143) centre (-511.1651, -152.4) ccw
  arc A9 (-559.8475, -166.9143) -> (559.8475, -166.9143) centre (0, 0) ccw
  circle A10 centre (0, 0) radius 158.75
  dimension "d46" = 317.5
  constraint coincident A4.centre A9.centre
  measures "d46" diameter of A10
extrude "Extrude6" add sketch "Sketch7" along normal blind 127 contours A10
mirror "Mirror1" about plane through (2565.4, 0, 0) normal (1, 0, 0) of bodies 1 merged
